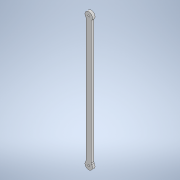
# Autodesk Inventor part: arm
Saved by Autodesk Inventor 2020 (Build 240168000, 168)
## iProperties
Created: 2020-03-17
Part Number: arm
Material: Generic
Document SubType Name: Modeling
Designer: erwin
Density: 1 g/cm^3
Appearance: Default
Author: erwin
Autodesk Inventor part; units mm, degrees
ref_plane "YZ Plane" through (0, 0, 0) normal (1, 0, 0) x (0, 1, 0)
ref_plane "XZ Plane" through (0, 0, 0) normal (0, 1, 0) x (-1, 0, 0)
ref_plane "XY Plane" through (0, 0, 0) normal (0, 0, 1) x (1, 0, 0)
ref_plane "Work Plane1" through (0, 0, 0) normal (0, 0, 1) x (1, 0, 0)
sketch "Sketch1" plane through (0, 0, 0) normal (0, 0, 1) x (1, 0, 0)
  arc A0 (-12, 16) -> (-12, 24) centre (-12, 20) ccw projected
  line L0 (-12, 3) -> (-12, 16) projected
  line L1 (0, 3) -> (-12, 3) projected
  line L2 (0, 3) -> (0, 30) projected
  line L3 (-12, 30) -> (0, 30) projected
  line L4 (-12, 24) -> (-12, 30) projected
  circle A1 centre (-12, 20) radius 4
  circle A2 centre (-12, 20) radius 17.5
  line L5 (-12, 20) -> (0, 20)
  line L6 (0, 20) -> (0, 320)
  line L7 (0, 320) -> (-12, 320)
  line L8 (-12, 320) -> (-12, 20)
  line L9 (-12, 320) -> (-24, 320)
  line L10 (-24, 320) -> (-24, 20)
  line L11 (-24, 20) -> (-12, 20)
  line L12 (-12, 20) -> (-12, 320)
  point P0 (0, 0)
  point P1 (0, 32.7377)
  point P2 (-24, 32.7377)
  dimension "d0" = 35
  dimension "d1" = 300
  dimension "d2" = 12
  constraints: 16 end point, 4 parallel, 2 coincident, 2 horizontal, 2 perpendicular, 1 centre point, 3 other
  measures "d0" diameter of A2
  measures "d1" distance of L6.end L5.end
  measures "d2" distance of L11.end L10.end
extrude "Extrusion1" add sketch "Sketch1" along normal blind 12 contours A0 L5 L2 A2 L1 L0 | L0 L1 A2 L10 L11 A1 | A0 L4 L3 L2 L5 | L11 L10 A2 L8 L4 A1 | L2 L6 A2 | L8 A2 L6 L3 | L10 L9 L8 A2 | L8 L7 L6 A2
fillet "Fillet1" radius 10 2 edges at (-24, 32.7377, 6) (0, 32.7377, 6)
mirror "Mirror1" about plane through (0, 320, 0) normal (0, 1, 0) of "Extrusion1"
body "Solid1"
